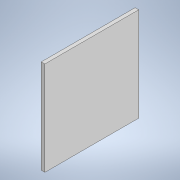
# Autodesk Inventor part: ogniwo_sloneczne
Saved by Autodesk Inventor 2021 (Build 250183000, 183)
## iProperties
Created: 2025-11-29
Part Number: ogniwo_sloneczne
Material: Generic
Document SubType Name: Modeling
Designer: huber
Density: 1 g/cm^3
Appearance: Default
Author: huber
Autodesk Inventor part; units mm, degrees
ref_plane "YZ Plane" through (0, 0, 0) normal (1, 0, 0) x (0, 1, 0)
ref_plane "XZ Plane" through (0, 0, 0) normal (0, 1, 0) x (-1, 0, 0)
ref_plane "XY Plane" through (0, 0, 0) normal (0, 0, 1) x (1, 0, 0)
sketch "Sketch1" plane through (0, 0, 0) normal (1, 0, 0) x (0, 1, 0)
  line L0 (32.5, 32.5) -> (-32.5, 32.5)
  line L1 (-32.5, 32.5) -> (-32.5, -32.5)
  line L2 (-32.5, -32.5) -> (32.5, -32.5)
  line L3 (32.5, -32.5) -> (32.5, 32.5)
  line L4 (32.5, 32.5) -> (-32.5, -32.5) construction
  line L5 (-32.5, 32.5) -> (32.5, -32.5) construction
  point P0 (0, 0)
  dimension "d0" = 65
  dimension "d1" = 65
  constraints: 12 end point, 2 midpoint, 2 parallel, 1 horizontal, 1 perpendicular
  measures "d0" distance of L1.end L2.end
  measures "d1" distance of L0.end L1.end
extrude "Extrusion1" add sketch "Sketch1" along normal blind 2.5
equation "\"d1\" = d0"
body "Solid1"
